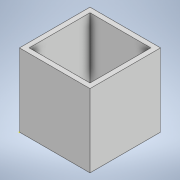
# Autodesk Inventor part: waterBallonHolderv2
Saved by Autodesk Inventor 2020.5 (Build 245400000, 400)
## iProperties
Created: 2022-09-14
Part Number: waterBallonHolderv2
Material: Generic
Document SubType Name: Sheet Metal
Designer: kouda
Density: 1 g/cm^3
Appearance: Default
Sheet Metal Rule: Default
Author: kouda
Autodesk Inventor part; units mm, degrees
ref_plane "YZ Plane" through (0, 0, 0) normal (1, 0, 0) x (0, 1, 0)
ref_plane "XZ Plane" through (0, 0, 0) normal (0, 1, 0) x (-1, 0, 0)
ref_plane "XY Plane" through (0, 0, 0) normal (0, 0, 1) x (1, 0, 0)
sketch "Sketch7" plane through (0, 0, 0) normal (0, 1, 0) x (-1, 0, 0)
  point P0 (0, 0)
sketch "Sketch8" plane through (0, 0, 0) normal (0, 1, 0) x (-1, 0, 0)
  line L0 (0, 0) -> (-29, 0)
  line L1 (-29, 0) -> (-29, -29)
  line L2 (-29, -29) -> (0, -29)
  line L3 (0, -29) -> (0, 0)
  line L4 (-2, -27) -> (-27, -27)
  line L5 (-27, -27) -> (-27, -2)
  line L6 (-27, -2) -> (-2, -2)
  line L7 (-2, -2) -> (-2, -27)
  dimension "d25" = 29
  dimension "d26" = 29
  dimension "d38" = 2
  constraints: 16 end point, 4 parallel, 2 perpendicular, 1 horizontal, 3 other
  measures "d25" distance of L2.end L1.end
  measures "d26" distance of L1.end L0.end
  measures "d38" distance between parallel lines of L2 L4
extrude "Extrusion5" add sketch "Sketch8" along normal blind 30 contours L3 L2 L1 L0 | L4 L5 L6 L7
sketch "Sketch11" plane through (0, 30, 0) normal (0, 1, 0) x (1, 0, 0)
  line L0 (0, 0) -> (29, 0) projected
  line L1 (29, 0) -> (29, 29) projected
  line L2 (29, 29) -> (0, 29) projected
  line L3 (0, 29) -> (0, 0) projected
  line L4 (2, 27) -> (27, 27)
  line L5 (27, 27) -> (27, 2)
  line L6 (27, 2) -> (2, 2)
  line L7 (2, 2) -> (2, 27)
  dimension "d39" = 2
  constraints: 8 end point, 3 other
  measures "d39" distance between parallel lines of L2 L4
extrude "Extrusion8" cut sketch "Sketch11" against normal blind 28 contours L4 L5 L6 L7
equation "\"BendRadius\" = Thickness"
equation "\"BendReliefWidth\" = Thickness"
equation "\"BendReliefDepth\" = 0.5 * Thickness"
equation "\"CornerReliefSize\" = 4 * Thickness"
equation "\"MinimumRemnant\" = 2 * Thickness"
equation "\"TransitionRadius\" = BendRadius"
equation "\"JacobiRadiusSize\" = Thickness"
equation "\"GapSize\" = Thickness"
equation "\"Thickness\" = 0.5"
body "Solid2"
